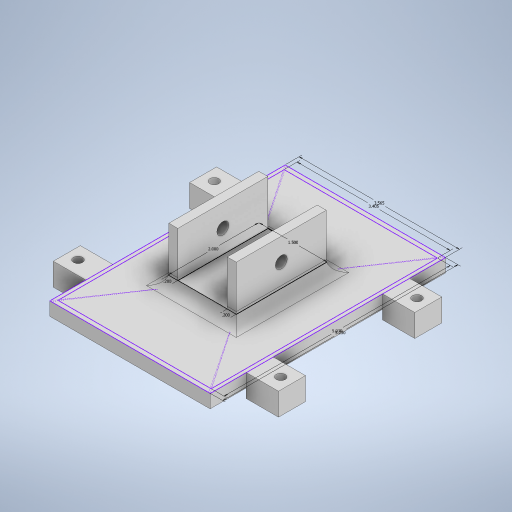
# Autodesk Inventor part: HotplateRetainer for 8020
Saved by Autodesk Inventor 2024.1 (Build 281209000, 209)
## iProperties
Created: 2022-02-14
Part Number: HotplateRetainer for 8020
Material: Generic
Document SubType Name: Modeling
Designer: Beaucage
Density: 1 g/cm^3
Appearance: Default
Author: Beaucage
Autodesk Inventor part; units mm, degrees
ref_plane "YZ Plane" through (0, 0, 0) normal (1, 0, 0) x (0, 1, 0)
ref_plane "XZ Plane" through (0, 0, 0) normal (0, 1, 0) x (-1, 0, 0)
ref_plane "XY Plane" through (0, 0, 0) normal (0, 0, 1) x (1, 0, 0)
sketch "Sketch1" plane through (0, 0, 0) normal (0, 1, 0) x (-1, 0, 0)
  line L0 (0, 0) -> (38.1, 0)
  line L1 (38.1, 0) -> (38.1, -50.8)
  line L2 (38.1, -50.8) -> (0, -50.8)
  line L3 (0, -50.8) -> (0, 0)
  line L4 (38.1, -50.8) -> (33.02, -50.8)
  line L5 (33.02, -50.8) -> (33.02, 0)
  line L6 (33.02, 0) -> (38.1, 0)
  line L7 (38.1, 0) -> (38.1, -50.8)
  line L8 (0, -50.8) -> (5.08, -50.8)
  line L9 (5.08, -50.8) -> (5.08, 0)
  line L10 (5.08, 0) -> (0, 0)
  line L11 (0, 0) -> (0, -50.8)
  dimension "d0" = 38.1
  dimension "d1" = 50.8
  dimension "d2" = 5.08
  dimension "d3" = 5.08
  constraints: 24 end point, 6 parallel, 3 horizontal, 3 perpendicular, 2 point on line
  measures "d0" distance of L1.end L2.end
  measures "d1" distance of L0.end L1.end
  measures "d2" distance of L5.end L6.end
  measures "d3" distance of L10.end L9.end
extrude "Extrusion1" add sketch "Sketch1" along normal blind 25.4 contours L0 L9 L2 L3 | L0 L1 L2 L5
extrude "Extrusion2" add sketch "Sketch1" against normal blind 5.08
sketch "Sketch2" plane through (0, 25.4, 0) normal (1, 0, 0) x (0, 0, -1)
  line L0 (50.8, 0) -> (0, 0) projected
  line L1 (25.4, 0) -> (25.4, -12.7)
  point P0 (0, -25.4)
  dimension "d8" = 12.7
  constraints: 2 end point, 1 midpoint, 1 vertical
  measures "d8" distance of L1.start L1.end
hole "Hole1" at (0, 12.7, -25.4) direction (-1, 0, 0) diameter 6.7564 end through all clearance for "Socket Head Cap Screw" size "1/4" standard "Ansi Unified Screw Threads"
sketch "Sketch3" plane through (0, -5.08, 0) normal (0, -1, 0) x (1, 0, 0)
  line L0 (0, 0) -> (-38.1, 0) projected
  line L1 (-38.1, 0) -> (-38.1, -50.8) projected
  line L2 (-38.1, -50.8) -> (0, -50.8) projected
  line L3 (0, -50.8) -> (0, 0) projected
  line L4 (-62.2986, 38.4797) -> (24.1986, 38.4797)
  line L5 (24.1986, 38.4797) -> (24.1986, -89.2797)
  line L6 (24.1986, -89.2797) -> (-62.2986, -89.2797)
  line L7 (-62.2986, -89.2797) -> (-62.2986, 38.4797)
  line L8 (-62.2986, 38.4797) -> (24.1986, -89.2797) construction
  line L9 (24.1986, 38.4797) -> (-62.2986, -89.2797) construction
  line L10 (-63.4909, 41.021) -> (25.3909, 41.021)
  line L11 (25.3909, -91.821) -> (-63.4909, -91.821)
  line L12 (-63.4909, 41.021) -> (25.3909, -91.821) construction
  line L13 (25.3909, 41.021) -> (-63.4909, -91.821) construction
  line L14 (-64.3255, 41.021) -> (26.2255, 41.021)
  line L15 (26.2255, 41.021) -> (26.2255, -91.821)
  line L16 (26.2255, -91.821) -> (-64.3255, -91.821)
  line L17 (-64.3255, -91.821) -> (-64.3255, 41.021)
  line L18 (-64.3255, 41.021) -> (26.2255, -91.821) construction
  line L19 (26.2255, 41.021) -> (-64.3255, -91.821) construction
  point P0 (-19.05, -25.4)
  point P1 (25.3909, 41.021)
  dimension "d16" = 86.4972
  dimension "d17" = 127.7595
  dimension "d18" = 132.842
  dimension "d19" = 90.551
  constraints: 32 end point, 6 midpoint, 5 parallel, 3 horizontal, 2 perpendicular
  measures "d16" distance of L5.end L6.end
  measures "d17" distance of L4.end L5.end
  measures "d18" distance of L10.end L11.start
  measures "d19" distance of L15.end L16.end
extrude "Extrusion3" add sketch "Sketch3" along normal blind 2.54 contours L3 L2 L1 L0 | L4 L5 L6 L7
extrude "Extrusion4" add sketch "Sketch3" along normal blind 7.62 contours L10 L14 L15 L16 L11 L17
fillet "Fillet1" radius 6.35 4 edges at (-38.1, -5.08, -25.4) (-19.05, -5.08, -50.8) (0, -5.08, -25.4) (-19.05, -5.08, 0)
sketch "Sketch4" plane through (0, -5.08, 0) normal (0, 1, 0) x (1, 0, 0)
  line L0 (-51.6255, 19.05) -> (-77.0255, 19.05)
  line L1 (-77.0255, 19.05) -> (-77.0255, 31.75)
  line L2 (-77.0255, 31.75) -> (-51.6255, 31.75)
  line L3 (-51.6255, 31.75) -> (-51.6255, 19.05)
  line L4 (-64.3255, -41.021) -> (-64.3255, 91.821) projected
  line L5 (-51.6255, 19.05) -> (-77.0255, 31.75) construction
  line L6 (-77.0255, 19.05) -> (-51.6255, 31.75) construction
  line L7 (13.5255, 19.05) -> (38.9255, 19.05)
  line L8 (38.9255, 19.05) -> (38.9255, 31.75)
  line L9 (38.9255, 31.75) -> (13.5255, 31.75)
  line L10 (13.5255, 31.75) -> (13.5255, 19.05)
  line L11 (26.2255, 91.821) -> (26.2255, -41.021) projected
  line L12 (13.5255, 19.05) -> (38.9255, 31.75) construction
  line L13 (38.9255, 19.05) -> (13.5255, 31.75) construction
  line L14 (24.1986, -38.4797) -> (24.1986, 89.2797) projected
  line L15 (24.1986, -38.4797) -> (24.1986, -13.0797)
  line L16 (-62.2986, -38.4797) -> (24.1986, -38.4797) projected
  line L17 (-62.2986, -38.4797) -> (-62.2986, -13.0797)
  line L18 (24.1986, 89.2797) -> (24.1986, 63.8797)
  line L19 (24.1986, 89.2797) -> (49.5986, 89.2797) construction
  line L20 (-62.2986, 89.2797) -> (-62.2986, 63.8797)
  line L21 (-62.2986, 89.2797) -> (-62.2986, -38.4797) projected
  line L22 (44.5186, -20.6997) -> (3.8786, -20.6997)
  line L23 (3.8786, -20.6997) -> (3.8786, -5.4597)
  line L24 (3.8786, -5.4597) -> (44.5186, -5.4597)
  line L25 (44.5186, -5.4597) -> (44.5186, -20.6997)
  line L26 (44.5186, -20.6997) -> (3.8786, -5.4597) construction
  line L27 (3.8786, -20.6997) -> (44.5186, -5.4597) construction
  line L28 (3.8786, 56.2597) -> (44.5186, 56.2597)
  line L29 (44.5186, 56.2597) -> (44.5186, 71.4997)
  line L30 (44.5186, 71.4997) -> (3.8786, 71.4997)
  line L31 (3.8786, 71.4997) -> (3.8786, 56.2597)
  line L32 (3.8786, 56.2597) -> (44.5186, 71.4997) construction
  line L33 (44.5186, 56.2597) -> (3.8786, 71.4997) construction
  line L34 (-41.9786, -20.6997) -> (-82.6186, -20.6997)
  line L35 (-82.6186, -20.6997) -> (-82.6186, -5.4597)
  line L36 (-82.6186, -5.4597) -> (-41.9786, -5.4597)
  line L37 (-41.9786, -5.4597) -> (-41.9786, -20.6997)
  line L38 (-41.9786, -20.6997) -> (-82.6186, -5.4597) construction
  line L39 (-82.6186, -20.6997) -> (-41.9786, -5.4597) construction
  line L40 (-41.9786, 56.2597) -> (-82.6186, 56.2597)
  line L41 (-82.6186, 56.2597) -> (-82.6186, 71.4997)
  line L42 (-82.6186, 71.4997) -> (-41.9786, 71.4997)
  line L43 (-41.9786, 71.4997) -> (-41.9786, 56.2597)
  line L44 (-41.9786, 56.2597) -> (-82.6186, 71.4997) construction
  line L45 (-82.6186, 56.2597) -> (-41.9786, 71.4997) construction
  point P0 (0, 0)
  point P1 (-64.3255, 25.4)
  point P2 (26.2255, 25.4)
  point P3 (26.2255, 31.75)
  point P4 (26.2255, 19.05)
  point P5 (-64.3255, 19.05)
  point P6 (-64.3255, 31.75)
  point P7 (-64.3255, -20.6997)
  point P8 (-64.3255, -5.4597)
  point P9 (-64.3255, 56.2597)
  point P10 (-64.3255, 71.4997)
  point P11 (26.2255, 71.4997)
  point P12 (26.2255, 56.2597)
  point P13 (26.2255, -5.4597)
  point P14 (26.2255, -20.6997)
  dimension "d25" = 25.4
  dimension "d26" = 12.7
  dimension "d27" = 25.4
  dimension "d28" = 12.7
  dimension "d38" = 25.4
  dimension "d39" = 25.4
  dimension "d40" = 25.4
  dimension "d41" = 90
  dimension "d42" = 25.4
  dimension "d43" = 40.64
  dimension "d44" = 15.24
  dimension "d45" = 40.64
  dimension "d46" = 15.24
  dimension "d47" = 40.64
  dimension "d48" = 15.24
  dimension "d49" = 40.64
  dimension "d50" = 15.24
  constraints: 82 end point, 14 midpoint, 13 parallel, 7 horizontal, 7 perpendicular, 2 point on line, 1 collinear
  measures "d25" distance of L1.end L2.end
  measures "d26" distance of L0.end L1.end
  measures "d27" distance of L9.end L8.end
  measures "d28" distance of L8.end L7.end
  measures "d38" distance of L14.start L15.end
  measures "d39" distance of L16.start L17.end
  measures "d40" distance of L14.end L18.end
  measures "d41" angle of L18 L19
  measures "d42" distance of L20.start L20.end
  measures "d43" distance of L23.end L24.end
  measures "d44" distance of L22.end L23.end
  measures "d45" distance of L30.end L29.end
  measures "d46" distance of L29.end L28.end
  measures "d47" distance of L35.end L36.end
  measures "d48" distance of L34.end L35.end
  measures "d49" distance of L41.end L42.end
  measures "d50" distance of L40.end L41.end
extrude "Extrusion5" add sketch "Sketch4" against normal blind 12.7 contours L4 L34 L35 L36 | L40 L41 L42 L4 | L24 L25 L22 L11 | L11 L30 L29 L28
sketch "Sketch6" plane through (0, -17.78, 0) normal (0, -1, 0) x (1, 0, 0)
  line L0 (-82.6186, -71.4997) -> (-82.6186, -56.2597) projected
  line L1 (-82.6186, -63.8797) -> (-62.2986, -63.8797)
  line L2 (-62.2986, -89.2797) -> (-62.2986, 38.4797) projected
  line L3 (-62.2986, -63.8797) -> (-76.2686, -63.8797)
  line L4 (24.1986, 38.4797) -> (24.1986, -89.2797) projected
  line L5 (-82.6186, 20.6997) -> (-82.6186, 5.4597) projected
  line L6 (44.5186, 5.4597) -> (44.5186, 20.6997) projected
  line L7 (44.5186, -71.4997) -> (44.5186, -56.2597) projected
  line L8 (44.5186, 13.0797) -> (38.1686, 13.0797)
  line L9 (44.5186, -63.8797) -> (38.1686, -63.8797)
  line L10 (-82.6186, 13.0797) -> (-76.2686, 13.0797)
  point P0 (0, 0)
  dimension "d51" = 13.97
  dimension "d52" = 6.35
  dimension "d53" = 6.35
  dimension "d54" = 6.35
  constraints: 10 end point, 4 midpoint, 3 horizontal, 2 point on line, 1 perpendicular
  measures "d51" distance of L1.end L3.end
  measures "d52" distance of L8.start L8.end
  measures "d53" distance of L9.start L9.end
  measures "d54" distance of L10.start L10.end
hole "Hole3" at (38.1686, -17.78, 13.0797) at (38.1686, -17.78, -63.8797) at (-76.2686, -17.78, -63.8797) at (-76.2686, -17.78, 13.0797) direction (0, 1, 0) diameter 5.1594 end through all
body "Solid1"
